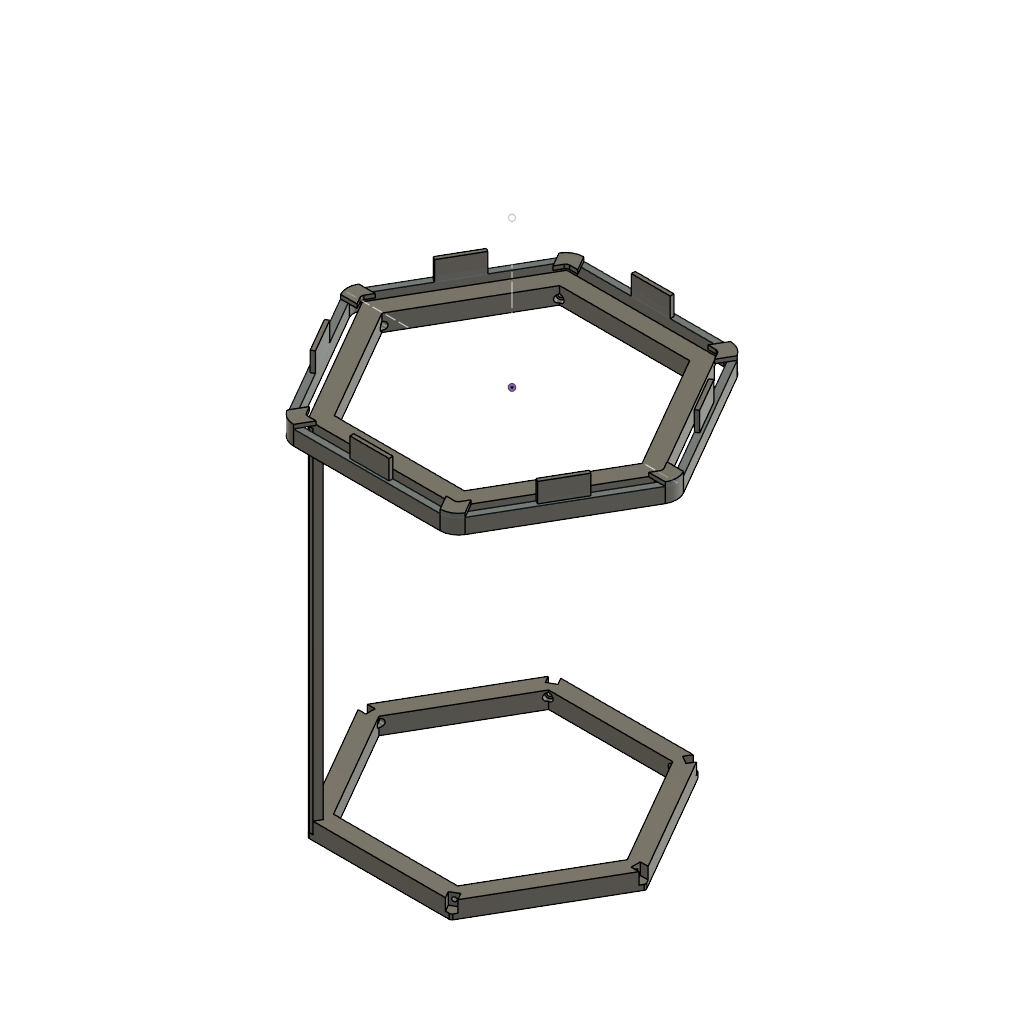
Transparent_PCB_Support (Autodesk Fusion 360 design; units mm, degrees)
Autodesk Fusion 360 part; units mm, degrees
sketch "Sketch1" plane through (0, 0, 0) normal (0, 1, 0) x (1, 0, 0) in component "TopHex"
  line L0 (0, 0) -> (114.9, 0)
  line L1 (114.9, 0) -> (172.35, 99.5063)
  line L2 (172.35, 99.5063) -> (114.9, 199.0126)
  line L3 (114.9, 199.0126) -> (0, 199.0126)
  line L4 (0, 199.0126) -> (-57.45, 99.5063)
  line L5 (-57.45, 99.5063) -> (0, 0)
  line L6 (-42.4389, 99.5063) -> (7.5056, 13)
  line L7 (7.5056, 13) -> (107.3944, 13)
  line L8 (107.3944, 13) -> (157.3389, 99.5063)
  line L9 (157.3389, 99.5063) -> (107.3944, 186.0126)
  line L10 (107.3944, 186.0126) -> (7.5056, 186.0126)
  line L11 (7.5056, 186.0126) -> (-42.4389, 99.5063)
  point P0 (57.45, 99.5063)
  dimension "d1" = 114.9
  dimension "d2" = -13
  constraint coincident L0.start L5.end
  measures "d1" distance of L0.start L0.end
extrude "Extrude1" add sketch "Sketch1" along normal blind 13 makes body 1 in component "TopHex"
ref_plane "WorkPlane1" through (114.9, 6.5, 0) normal (0.5, 0, 0.866025) x (0, 1, 0) in component "TopHex"
sketch "Sketch2" plane through (28.725, 0, 49.7532) normal (0.5, 0, 0.866025) x (0, 1, 0) in component "TopHex"
  line L0 (0, 0) -> (0, -99.5063) construction
  line L1 (0, -99.5063) -> (13, -99.5063) construction
  line L2 (13, -99.5063) -> (13, 0) construction
  line L3 (13, 0) -> (0, 0) construction
  line L4 (0, -99.5063) -> (0, -199.0126) construction
  line L5 (0, -199.0126) -> (13, -199.0126) construction
  line L6 (13, -199.0126) -> (13, -99.5063) construction
  line L7 (13, -99.5063) -> (0, -99.5063) construction
  line L8 (0, -99.5063) -> (9, -99.5063) construction
  line L9 (9, -103.0063) -> (0, -103.0063)
  line L10 (0, -103.0063) -> (0, -96.0063)
  line L11 (0, -96.0063) -> (9, -96.0063)
  line L12 (9, -96.0063) -> (9, -103.0063)
  line L13 (9, -103.0063) -> (0, -96.0063) construction
  line L14 (0, -103.0063) -> (9, -96.0063) construction
  point P0 (4.5, -99.5063)
  dimension "d6" = 9
  dimension "d7" = 7
  constraint coincident L0.end L1.start
  constraint perpendicular L4 L8
  constraint horizontal L9
  constraint perpendicular L9 L10
  constraint parallel L9 L11
  constraint parallel L10 L12
  constraint coincident L13 P0
  constraint coincident L14 P0
  constraint midpoint L8 P0
  constraint collinear L0 L10
  measures "d6" distance of L0.end L8.end
  measures "d7" distance of L9.end L10.end
extrude "Extrude2" cut sketch "Sketch2" against normal blind 8 bodies 1 in component "TopHex"
fillet "Fillet1" radius 2 1 edges at (114.9, 11, 0) on bodies 1 in component "TopHex"
sketch "Sketch3" plane through (24.725, 0, 42.825) normal (0.5, 0, 0.866025) x (0.866025, 0, -0.5) in component "TopHex"
  line L0 (96.0063, 9) -> (96.0063, 0)
  line L1 (96.0063, 0) -> (103.0063, 0)
  line L2 (103.0063, 0) -> (103.0063, 9)
  line L3 (103.0063, 9) -> (96.0063, 9)
  line L4 (96.0063, 9) -> (103.0063, 0) construction
  line L5 (96.0063, 0) -> (103.0063, 9) construction
  circle A0 centre (99.5063, 4.5) radius 1.6
  dimension "d12" = 3.2
  constraint coincident L0.start L3.end
  constraint coincident L1.end L2.start
  constraint coincident L0.end L1.start
  constraint coincident L2.end L3.start
  constraint midpoint L5 A0.centre
  measures "d12" diameter of A0
extrude "Extrude3" cut sketch "Sketch3" against normal blind 8.5 contours A0 bodies 1 in component "TopHex"
sketch "Sketch4" plane through (24.725, 0, 42.825) normal (0.5, 0, 0.866025) x (0.866025, 0, -0.5) in component "TopHex"
  circle A0 centre (99.5063, 4.5) radius 1.6
  line L0 (96.0063, 9) -> (96.0063, 0)
  line L1 (96.0063, 0) -> (103.0063, 0)
  line L2 (103.0063, 0) -> (103.0063, 9)
  line L3 (103.0063, 9) -> (96.0063, 9)
  circle A1 centre (99.5063, 4.5) radius 1.6 construction
  circle A2 centre (99.5063, 4.5) radius 3
  dimension "d15" = 6
  constraint concentric A1 A2
  measures "d15" diameter of A2
extrude "Extrude4" cut sketch "Sketch4" against normal blind 5 from surface at -4 contours A0 | A2 bodies 1 in component "TopHex"
sketch "Sketch5" plane through (0, 0, 0) normal (0, 1, 0) x (1, 0, 0) in component "TopHex"
  arc A0 (113.7453, 0) -> (115.4774, 1) centre (113.7453, 2) ccw construction
  line L0 (115.4774, 1) -> (172.35, 99.5063) construction
  line L1 (172.35, 99.5063) -> (114.9, 199.0126) construction
  line L2 (114.9, 199.0126) -> (0, 199.0126) construction
  line L3 (0, 199.0126) -> (-57.45, 99.5063) construction
  line L4 (-57.45, 99.5063) -> (0, 0) construction
  line L5 (0, 0) -> (113.7453, 0) construction
  line L6 (-42.4389, 99.5063) -> (7.5056, 186.0126) construction
  line L7 (7.5056, 186.0126) -> (107.3944, 186.0126) construction
  line L8 (107.3944, 186.0126) -> (157.3389, 99.5063) construction
  line L9 (157.3389, 99.5063) -> (107.3944, 13) construction
  line L10 (107.3944, 13) -> (7.5056, 13) construction
  line L11 (7.5056, 13) -> (-42.4389, 99.5063) construction
  line L12 (0, 0) -> (114.9, 199.0126) construction
  line L13 (0, 199.0126) -> (107.3944, 13) construction
  constraint coincident L4.end L5.start
  constraint coincident L1.end L2.start
  constraint coincident L2.end L3.start
  constraint coincident L9.end L10.start
ref_plane "WorkPlane2" through (57.45, 0, -99.5063) normal (0.5, 0, -0.866025) x (0, 1, 0) in component "TopHex"
sketch "Sketch6" plane through (57.45, 0, -99.5063) normal (0.5, 0, -0.866025) x (0, 1, 0) in component "TopHex"
  line L0 (0, 0) -> (113, 0)
  constraint coincident L0.start origin
  constraint horizontal L0
pattern_circular "C-Pattern1" count 6 over 360 about axis through (57.45, 0, -99.5063) along (0, 1, 0) of "Extrude2", "Extrude3", "Extrude4" in component "TopHex"
fillet "Fillet2" radius 2 5 edges at (172.35, 11, -99.5063) (114.9, 11, -199.0126) (0, 11, -199.0126) (-57.45, 11, -99.5063) (0, 11, 0) on bodies 1 in component "TopHex"
ref_plane "WorkPlane1" through (57.45, -265, -99.5063) normal (0, 1, 0) x (0, 0, 1) in component "BottomHex"
sketch "Sketch1 (2)" plane through (0, -265, 0) normal (0, 1, 0) x (1, 0, 0) in component "BottomHex"
  line L0 (0, 0) -> (109.9, 0)
  line L1 (109.9, 0) -> (164.85, 95.1762)
  line L2 (164.85, 95.1762) -> (109.9, 190.3524)
  line L3 (109.9, 190.3524) -> (0, 190.3524)
  line L4 (0, 190.3524) -> (-54.95, 95.1762)
  line L5 (-54.95, 95.1762) -> (0, 0)
  line L6 (7.2746, 12.6) -> (102.6254, 12.6)
  line L7 (102.6254, 12.6) -> (150.3008, 95.1762)
  line L8 (150.3008, 95.1762) -> (102.6254, 177.7524)
  line L9 (102.6254, 177.7524) -> (7.2746, 177.7524)
  line L10 (7.2746, 177.7524) -> (-40.4008, 95.1762)
  line L11 (-40.4008, 95.1762) -> (7.2746, 12.6)
  point P0 (54.95, 95.1762)
  dimension "d26" = 109.9
  dimension "d27" = -12.6
  constraint coincident L0.start L5.end
  measures "d26" distance of L0.start L0.end
extrude "Extrude1'" add sketch "Sketch1 (2)" along normal blind 13 separate body makes body 2 in component "BottomHex"
ref_plane "WorkPlane2" through (0, -258.5, 0) normal (-0.5, 0, 0.866025) x (0, 1, 0) in component "BottomHex"
sketch "Sketch2 (2)" plane through (0, 0, 0) normal (-0.5, 0, 0.866025) x (0, 1, 0) in component "BottomHex"
  line L0 (-265, 0) -> (-252, 0) construction
  line L1 (-265, 95.1762) -> (-265, 0) construction
  line L2 (-265, 0) -> (-252, 0) construction
  line L3 (-252, 0) -> (-252, 95.1762) construction
  line L4 (-252, 95.1762) -> (-265, 95.1762) construction
  line L5 (-265, 0) -> (-265, -95.1762) construction
  line L6 (-265, -95.1762) -> (-252, -95.1762) construction
  line L7 (-252, -95.1762) -> (-252, 0) construction
  line L8 (-252, 0) -> (-265, 0) construction
  line L9 (-252, 0) -> (-261, 0) construction
  line L10 (-252, -3.5) -> (-261, -3.5)
  line L11 (-261, -3.5) -> (-261, 3.5)
  line L12 (-261, 3.5) -> (-252, 3.5)
  line L13 (-252, 3.5) -> (-252, -3.5)
  line L14 (-252, -3.5) -> (-261, 3.5) construction
  line L15 (-261, -3.5) -> (-252, 3.5) construction
  point P0 (-256.5, 0)
  dimension "d31" = 9
  dimension "d32" = 9
  dimension "d33" = 7
  constraint coincident L0.end L2.end
  constraint perpendicular L3 L9
  constraint horizontal L10
  constraint perpendicular L10 L11
  constraint parallel L10 L12
  constraint parallel L11 L13
  constraint coincident L14 P0
  constraint coincident L15 P0
  constraint midpoint L9 P0
  measures "d31" distance of L0.end L9.end
  measures "d32" distance of L11.end L12.end
  measures "d33" distance of L10.end L11.end
extrude "Extrude2'" cut sketch "Sketch2 (2)" against normal blind 8 bodies 2 in component "BottomHex"
sketch "Sketch3 (2)" plane through (4, 0, -6.9282) normal (-0.5, 0, 0.866025) x (0.866025, 0, 0.5) in component "BottomHex"
  line L0 (-3.5, -252) -> (-3.5, -261)
  line L1 (-3.5, -261) -> (3.5, -261)
  line L2 (3.5, -261) -> (3.5, -252)
  line L3 (3.5, -252) -> (-3.5, -252)
  line L4 (-3.5, -261) -> (3.5, -252) construction
  line L5 (-3.5, -252) -> (3.5, -261) construction
  circle A0 centre (0, -256.5) radius 1.6
  dimension "d36" = 3.2
  constraint coincident L0.end L1.start
  constraint coincident L2.end L3.start
  constraint coincident L0.start L3.end
  constraint coincident L1.end L2.start
  constraint midpoint L4 A0.centre
  measures "d36" diameter of A0
extrude "Extrude3'" cut sketch "Sketch3 (2)" against normal blind 10 contours A0 bodies 2 in component "BottomHex"
sketch "Sketch4 (2)" plane through (4, 0, -6.9282) normal (-0.5, 0, 0.866025) x (0.866025, 0, 0.5) in component "BottomHex"
  circle A0 centre (0, -256.5) radius 1.6
  line L0 (-3.5, -252) -> (-3.5, -261)
  line L1 (-3.5, -261) -> (3.5, -261)
  line L2 (3.5, -261) -> (3.5, -252)
  line L3 (3.5, -252) -> (-3.5, -252)
  circle A1 centre (0, -256.5) radius 1.6 construction
  circle A2 centre (0, -256.5) radius 3
  dimension "d39" = 6
  constraint concentric A1 A2
  measures "d39" diameter of A2
extrude "Extrude4'" cut sketch "Sketch4 (2)" against normal blind 5 from surface at -4 contours A2 bodies 2 in component "BottomHex"
sketch "Sketch5 (2)" plane through (0, -252, 0) normal (0, 1, 0) x (-1, 0, 0) in component "BottomHex"
  line L0 (2.0207, -3.5) -> (-0.9689, -8.6782)
  line L1 (-0.9689, -8.6782) -> (-7.0311, -5.1782)
  line L2 (-7.0311, -5.1782) -> (-4.0415, 0)
  line L3 (-4.0415, 0) -> (-109.9, 0)
  line L4 (-109.9, 0) -> (-164.85, -95.1762)
  line L5 (-164.85, -95.1762) -> (-109.9, -190.3524)
  line L6 (-109.9, -190.3524) -> (0, -190.3524)
  line L7 (0, -190.3524) -> (54.95, -95.1762)
  line L8 (54.95, -95.1762) -> (2.0207, -3.5)
  line L9 (-7.2746, -12.6) -> (40.4008, -95.1762)
  line L10 (40.4008, -95.1762) -> (-7.2746, -177.7524)
  line L11 (-7.2746, -177.7524) -> (-102.6254, -177.7524)
  line L12 (-102.6254, -177.7524) -> (-150.3008, -95.1762)
  line L13 (-150.3008, -95.1762) -> (-102.6254, -12.6)
  line L14 (-102.6254, -12.6) -> (-7.2746, -12.6)
  line L15 (-7.2746, -12.6) -> (-102.6254, -177.7524) construction
  constraint coincident L9.start L14.end
  constraint coincident L11.end L12.start
ref_plane "WorkPlane3" through (54.95, -252, -95.1762) normal (0.5, 0, -0.866025) x (0, 1, 0) in component "BottomHex"
sketch "Sketch6 (2)" plane through (54.95, -252, -95.1762) normal (0.5, 0, -0.866025) x (0, 1, 0) in component "BottomHex"
  line L0 (0, 0) -> (115, 0)
  constraint coincident L0.start origin
  constraint horizontal L0
pattern_circular "C-Pattern1'" count 6 over 360 about axis through (54.95, -252, -95.1762) along (0, 1, 0) of "Extrude2'", "Extrude3'", "Extrude4'" in component "BottomHex"
fillet "Fillet1'" radius 2 6 edges at (0, -263, 0) (109.9, -263, 0) (164.85, -263, -95.1762) (109.9, -263, -190.3524) (0, -263, -190.3524) (-54.95, -263, -95.1762) on bodies 2 in component "BottomHex"
sketch "Sketch1 (3)" plane through (0, 9, 0) normal (0, -1, 0) x (1, 0, 0) in component "Connection"
  line L0 (-2.0207, -3.5) -> (0.9689, -8.6782)
  line L1 (0.9689, -8.6782) -> (7.0311, -5.1782)
  line L2 (7.0311, -5.1782) -> (4.0415, 0)
  line L3 (-2.0207, -3.5) -> (0.9689, -8.6782) construction
  line L4 (7.0311, -5.1782) -> (4.0415, 0) construction
  line L5 (0.9689, -8.6782) -> (7.0311, -5.1782) construction
  arc A0 (1.1547, 0) -> (-0.5774, -1) centre (1.1547, -2) ccw construction
  line L6 (1.1547, 0) -> (108.7453, 0) construction
  line L7 (-1.8764, -3.45) -> (1.0238, -8.4733)
  line L8 (1.0238, -8.4733) -> (6.8262, -5.1233)
  line L9 (6.8262, -5.1233) -> (3.926, -0.1)
  line L10 (-54.3726, -94.1762) -> (-0.5774, -1) construction
  arc A1 (1.1547, -0.1) -> (-0.4907, -1.05) centre (1.1547, -2) ccw
  line L11 (1.1547, -0.1) -> (3.926, -0.1)
  line L12 (-1.8764, -3.45) -> (-0.4907, -1.05)
  constraint coincident L0.start L3.start
  constraint coincident L0.end L1.start
  constraint coincident L1.end L2.start
  constraint coincident L2.end L4.end
  constraint concentric A0 A1
  constraint tangent A1 L11
extrude "Extrude1''" add sketch "Sketch1 (3)" along normal blind 270 separate body makes body 3 in component "Connection"
sketch "Sketch2 (3)" plane through (3.925, 0, -6.7983) normal (0.5, 0, -0.866025) x (-0.866025, 0, -0.5) in component "Connection"
  line L0 (3.35, 9) -> (-3.35, 9)
  line L1 (-3.35, 9) -> (-3.35, -261)
  line L2 (-3.35, -261) -> (3.35, -261)
  line L3 (3.35, -261) -> (3.35, 9)
  circle A0 centre (0, 4.5) radius 1.6 construction
  circle A1 centre (0, -256.5) radius 1.6 construction
  circle A2 centre (0, -256.5) radius 1.475
  circle A3 centre (0, 4.5) radius 1.475
  dimension "d52" = 2.95
  dimension "d53" = 2.95
  constraint concentric A1 A2
  constraint concentric A0 A3
  measures "d52" diameter of A2
  measures "d53" diameter of A3
extrude "Extrude2''" cut sketch "Sketch2 (3)" against normal blind 6 contours A2 | A3 bodies 3 in component "Connection"
ref_plane "WorkPlane1" through (57.45, 10, -99.5063) normal (0, 1, 0) x (0, 0, 1) in component "OutsideSupport"
sketch "Sketch1 (4)" plane through (0, 10, 0) normal (0, 1, 0) x (1, 0, 0) in component "OutsideSupport"
  arc A0 (-0.5774, 1) -> (1.1547, 0) centre (1.1547, 2) ccw construction
  line L0 (1.1547, 0) -> (113.7453, 0) construction
  arc A1 (113.7453, 0) -> (115.4774, 1) centre (113.7453, 2) ccw construction
  line L1 (115.4774, 1) -> (171.7726, 98.5063) construction
  arc A2 (171.7726, 98.5063) -> (171.7726, 100.5063) centre (170.0406, 99.5063) ccw construction
  line L2 (171.7726, 100.5063) -> (115.4774, 198.0126) construction
  arc A3 (115.4774, 198.0126) -> (113.7453, 199.0126) centre (113.7453, 197.0126) ccw construction
  line L3 (113.7453, 199.0126) -> (1.1547, 199.0126) construction
  arc A4 (1.1547, 199.0126) -> (-0.5774, 198.0126) centre (1.1547, 197.0126) ccw construction
  line L4 (-0.5774, 198.0126) -> (-56.8726, 100.5063) construction
  arc A5 (-56.8726, 100.5063) -> (-56.8726, 98.5063) centre (-55.1406, 99.5063) ccw construction
  line L5 (-56.8726, 98.5063) -> (-0.5774, 1) construction
  line L6 (-42.4389, 99.5063) -> (7.5056, 186.0126) construction
  line L7 (7.5056, 186.0126) -> (107.3944, 186.0126) construction
  line L8 (107.3944, 186.0126) -> (157.3389, 99.5063) construction
  line L9 (157.3389, 99.5063) -> (107.3944, 13) construction
  line L10 (107.3944, 13) -> (7.5056, 13) construction
  line L11 (7.5056, 13) -> (-42.4389, 99.5063) construction
  line L12 (121.5395, -2.5) -> (177.8348, 95.0063)
  arc A6 (177.8348, 95.0063) -> (177.8348, 104.0063) centre (170.0406, 99.5063) ccw
  line L13 (177.8348, 104.0063) -> (121.5395, 201.5126)
  arc A7 (121.5395, 201.5126) -> (113.7453, 206.0126) centre (113.7453, 197.0126) ccw
  line L14 (113.7453, 206.0126) -> (1.1547, 206.0126)
  arc A8 (1.1547, 206.0126) -> (-6.6395, 201.5126) centre (1.1547, 197.0126) ccw
  line L15 (-6.6395, 201.5126) -> (-62.9348, 104.0063)
  arc A9 (-62.9348, 104.0063) -> (-62.9348, 95.0063) centre (-55.1406, 99.5063) ccw
  line L16 (-62.9348, 95.0063) -> (-6.6395, -2.5)
  arc A10 (-6.6395, -2.5) -> (1.1547, -7) centre (1.1547, 2) ccw
  line L17 (1.1547, -7) -> (113.7453, -7)
  arc A11 (113.7453, -7) -> (121.5395, -2.5) centre (113.7453, 2) ccw
  line L18 (125.8697, -5) -> (182.165, 92.5063)
  arc A12 (182.165, 92.5063) -> (182.165, 106.5063) centre (170.0406, 99.5063) ccw
  line L19 (182.165, 106.5063) -> (125.8697, 204.0126)
  arc A13 (125.8697, 204.0126) -> (113.7453, 211.0126) centre (113.7453, 197.0126) ccw
  line L20 (113.7453, 211.0126) -> (1.1547, 211.0126)
  arc A14 (1.1547, 211.0126) -> (-10.9697, 204.0126) centre (1.1547, 197.0126) ccw
  line L21 (-10.9697, 204.0126) -> (-67.265, 106.5063)
  arc A15 (-67.265, 106.5063) -> (-67.265, 92.5063) centre (-55.1406, 99.5063) ccw
  line L22 (-67.265, 92.5063) -> (-10.9697, -5)
  arc A16 (-10.9697, -5) -> (1.1547, -12) centre (1.1547, 2) ccw
  line L23 (1.1547, -12) -> (113.7453, -12)
  arc A17 (113.7453, -12) -> (125.8697, -5) centre (113.7453, 2) ccw
  dimension "d57" = 7
  dimension "d58" = 12
extrude "Extrude1'''" add sketch "Sketch1 (4)" against normal blind 8 separate body makes body 4 in component "OutsideSupport"
sketch "Sketch2 (4)" plane through (0, 10, 0) normal (0, 1, 0) x (-1, 0, 0) in component "OutsideSupport"
  arc A0 (-113.7453, 7) -> (-121.5395, 2.5) centre (-113.7453, -2) ccw
  line L0 (-113.7453, 7) -> (-1.1547, 7)
  arc A1 (6.6395, 2.5) -> (-1.1547, 7) centre (-1.1547, -2) ccw
  line L1 (6.6395, 2.5) -> (62.9348, -95.0063)
  arc A2 (62.9348, -104.0063) -> (62.9348, -95.0063) centre (55.1406, -99.5063) ccw
  line L2 (62.9348, -104.0063) -> (6.6395, -201.5126)
  arc A3 (-1.1547, -206.0126) -> (6.6395, -201.5126) centre (-1.1547, -197.0126) ccw
  line L3 (-1.1547, -206.0126) -> (-113.7453, -206.0126)
  arc A4 (-121.5395, -201.5126) -> (-113.7453, -206.0126) centre (-113.7453, -197.0126) ccw
  line L4 (-121.5395, -201.5126) -> (-177.8348, -104.0063)
  arc A5 (-177.8348, -95.0063) -> (-177.8348, -104.0063) centre (-170.0406, -99.5063) ccw
  line L5 (-177.8348, -95.0063) -> (-121.5395, 2.5)
  arc A6 (-113.7453, 12) -> (-125.8697, 5) centre (-113.7453, -2) ccw
  line L6 (-125.8697, 5) -> (-182.165, -92.5063)
  arc A7 (-182.165, -92.5063) -> (-182.165, -106.5063) centre (-170.0406, -99.5063) ccw
  line L7 (-182.165, -106.5063) -> (-125.8697, -204.0126)
  arc A8 (-125.8697, -204.0126) -> (-113.7453, -211.0126) centre (-113.7453, -197.0126) ccw
  line L8 (-113.7453, -211.0126) -> (-1.1547, -211.0126)
  arc A9 (-1.1547, -211.0126) -> (10.9697, -204.0126) centre (-1.1547, -197.0126) ccw
  line L9 (10.9697, -204.0126) -> (67.265, -106.5063)
  arc A10 (67.265, -106.5063) -> (67.265, -92.5063) centre (55.1406, -99.5063) ccw
  line L10 (67.265, -92.5063) -> (10.9697, 5)
  arc A11 (10.9697, 5) -> (-1.1547, 12) centre (-1.1547, -2) ccw
  line L11 (-1.1547, 12) -> (-113.7453, 12)
  line L12 (6.6395, 2.5) -> (62.9348, -95.0063) construction
  arc A12 (64.6669, -105.0063) -> (64.6669, -94.0063) centre (55.1406, -99.5063) ccw
  line L13 (8.3716, 3.5) -> (64.6669, -94.0063)
  arc A13 (8.3716, 3.5) -> (-1.1547, 9) centre (-1.1547, -2) ccw
  line L14 (-113.7453, 9) -> (-1.1547, 9)
  arc A14 (-113.7453, 9) -> (-123.2716, 3.5) centre (-113.7453, -2) ccw
  line L15 (-179.5669, -94.0063) -> (-123.2716, 3.5)
  arc A15 (-179.5669, -94.0063) -> (-179.5669, -105.0063) centre (-170.0406, -99.5063) ccw
  line L16 (-123.2716, -202.5126) -> (-179.5669, -105.0063)
  arc A16 (-123.2716, -202.5126) -> (-113.7453, -208.0126) centre (-113.7453, -197.0126) ccw
  line L17 (-1.1547, -208.0126) -> (-113.7453, -208.0126)
  arc A17 (-1.1547, -208.0126) -> (8.3716, -202.5126) centre (-1.1547, -197.0126) ccw
  line L18 (64.6669, -105.0063) -> (8.3716, -202.5126)
  dimension "d61" = -2
extrude "Extrude2'''" add sketch "Sketch2 (4)" along normal blind 3.5 contours A6 L6 A7 L7 A8 L8 A9 L9 A10 L10 A11 L11 | A12 L13 A13 L14 A14 L15 A15 L16 A16 L17 A17 L18 bodies 4 in component "OutsideSupport"
sketch "Sketch3 (3)" plane through (0, 13.5, 0) normal (0, 1, 0) x (-1, 0, 0) in component "OutsideSupport"
  line L0 (-1.1547, 12) -> (-113.7453, 12)
  arc A0 (-113.7453, 12) -> (-125.8697, 5) centre (-113.7453, -2) ccw
  line L1 (-125.8697, 5) -> (-182.165, -92.5063)
  arc A1 (-182.165, -92.5063) -> (-182.165, -106.5063) centre (-170.0406, -99.5063) ccw
  line L2 (-182.165, -106.5063) -> (-125.8697, -204.0126)
  arc A2 (-125.8697, -204.0126) -> (-113.7453, -211.0126) centre (-113.7453, -197.0126) ccw
  line L3 (-113.7453, -211.0126) -> (-1.1547, -211.0126)
  arc A3 (-1.1547, -211.0126) -> (10.9697, -204.0126) centre (-1.1547, -197.0126) ccw
  line L4 (10.9697, -204.0126) -> (67.265, -106.5063)
  arc A4 (67.265, -106.5063) -> (67.265, -92.5063) centre (55.1406, -99.5063) ccw
  line L5 (67.265, -92.5063) -> (10.9697, 5)
  arc A5 (10.9697, 5) -> (-1.1547, 12) centre (-1.1547, -2) ccw
  arc A6 (0.5774, -1) -> (-1.1547, 0) centre (-1.1547, -2) ccw construction
  line L6 (-1.1547, 0) -> (-113.7453, 0) construction
  arc A7 (-113.7453, 0) -> (-115.4774, -1) centre (-113.7453, -2) ccw construction
  line L7 (-115.4774, -1) -> (-171.7726, -98.5063) construction
  arc A8 (-171.7726, -98.5063) -> (-171.7726, -100.5063) centre (-170.0406, -99.5063) ccw construction
  line L8 (-171.7726, -100.5063) -> (-115.4774, -198.0126) construction
  arc A9 (-115.4774, -198.0126) -> (-113.7453, -199.0126) centre (-113.7453, -197.0126) ccw construction
  line L9 (-113.7453, -199.0126) -> (-1.1547, -199.0126) construction
  arc A10 (-1.1547, -199.0126) -> (0.5774, -198.0126) centre (-1.1547, -197.0126) ccw construction
  line L10 (0.5774, -198.0126) -> (56.8726, -100.5063) construction
  arc A11 (56.8726, -100.5063) -> (56.8726, -98.5063) centre (55.1406, -99.5063) ccw construction
  line L11 (56.8726, -98.5063) -> (0.5774, -1) construction
  line L12 (42.4389, -99.5063) -> (-7.5056, -186.0126) construction
  line L13 (-7.5056, -186.0126) -> (-107.3944, -186.0126) construction
  line L14 (-107.3944, -186.0126) -> (-157.3389, -99.5063) construction
  line L15 (-157.3389, -99.5063) -> (-107.3944, -13) construction
  line L16 (-107.3944, -13) -> (-7.5056, -13) construction
  line L17 (-7.5056, -13) -> (42.4389, -99.5063) construction
  line L18 (41.2842, -99.5063) -> (-8.0829, -185.0126)
  line L19 (-8.0829, -185.0126) -> (-106.8171, -185.0126)
  line L20 (-106.8171, -185.0126) -> (-156.1842, -99.5063)
  line L21 (-156.1842, -99.5063) -> (-106.8171, -14)
  line L22 (-106.8171, -14) -> (-8.0829, -14)
  line L23 (-8.0829, -14) -> (41.2842, -99.5063)
  arc A12 (-113.7453, 7) -> (-121.5395, 2.5) centre (-113.7453, -2) ccw
  line L24 (-121.5395, 2.5) -> (-177.8348, -95.0063)
  arc A13 (-177.8348, -95.0063) -> (-177.8348, -104.0063) centre (-170.0406, -99.5063) ccw
  line L25 (-177.8348, -104.0063) -> (-121.5395, -201.5126)
  arc A14 (-121.5395, -201.5126) -> (-113.7453, -206.0126) centre (-113.7453, -197.0126) ccw
  line L26 (-113.7453, -206.0126) -> (-1.1547, -206.0126)
  arc A15 (-1.1547, -206.0126) -> (6.6395, -201.5126) centre (-1.1547, -197.0126) ccw
  line L27 (6.6395, -201.5126) -> (62.9348, -104.0063)
  arc A16 (62.9348, -104.0063) -> (62.9348, -95.0063) centre (55.1406, -99.5063) ccw
  line L28 (62.9348, -95.0063) -> (6.6395, 2.5)
  arc A17 (6.6395, 2.5) -> (-1.1547, 7) centre (-1.1547, -2) ccw
  line L29 (-1.1547, 7) -> (-113.7453, 7)
  arc A18 (-113.7453, 12) -> (-125.8697, 5) centre (-113.7453, -2) ccw
  line L30 (-113.7453, 12) -> (-1.1547, 12)
  arc A19 (10.9697, 5) -> (-1.1547, 12) centre (-1.1547, -2) ccw
  line L31 (10.9697, 5) -> (67.265, -92.5063)
  arc A20 (67.265, -106.5063) -> (67.265, -92.5063) centre (55.1406, -99.5063) ccw
  line L32 (67.265, -106.5063) -> (10.9697, -204.0126)
  arc A21 (-1.1547, -211.0126) -> (10.9697, -204.0126) centre (-1.1547, -197.0126) ccw
  line L33 (-1.1547, -211.0126) -> (-113.7453, -211.0126)
  arc A22 (-125.8697, -204.0126) -> (-113.7453, -211.0126) centre (-113.7453, -197.0126) ccw
  line L34 (-125.8697, -204.0126) -> (-182.165, -106.5063)
  arc A23 (-182.165, -92.5063) -> (-182.165, -106.5063) centre (-170.0406, -99.5063) ccw
  line L35 (-182.165, -92.5063) -> (-125.8697, 5)
  arc A24 (-121.5395, -201.5126) -> (-113.7453, -206.0126) centre (-113.7453, -197.0126) ccw
  line L36 (-121.5395, -201.5126) -> (-177.8348, -104.0063)
  arc A25 (-177.8348, -95.0063) -> (-177.8348, -104.0063) centre (-170.0406, -99.5063) ccw
  line L37 (-177.8348, -95.0063) -> (-121.5395, 2.5)
  arc A26 (-113.7453, 7) -> (-121.5395, 2.5) centre (-113.7453, -2) ccw
  line L38 (-113.7453, 7) -> (-1.1547, 7)
  arc A27 (6.6395, 2.5) -> (-1.1547, 7) centre (-1.1547, -2) ccw
  line L39 (6.6395, 2.5) -> (62.9348, -95.0063)
  arc A28 (62.9348, -104.0063) -> (62.9348, -95.0063) centre (55.1406, -99.5063) ccw
  line L40 (62.9348, -104.0063) -> (6.6395, -201.5126)
  arc A29 (-1.1547, -206.0126) -> (6.6395, -201.5126) centre (-1.1547, -197.0126) ccw
  line L41 (-1.1547, -206.0126) -> (-113.7453, -206.0126)
  line L42 (-0.1547, -0.2679) -> (5.8453, 10.1244)
  line L43 (-1.1547, 12) -> (-8.0829, 0)
  line L44 (-116.3434, -0.5) -> (-172.6387, -98.0063)
  arc A30 (-172.6387, -98.0063) -> (-172.6387, -101.0063) centre (-170.0406, -99.5063) ccw
  line L45 (-172.6387, -101.0063) -> (-116.3434, -198.5126)
  arc A31 (-116.3434, -198.5126) -> (-113.7453, -200.0126) centre (-113.7453, -197.0126) ccw
  line L46 (-113.7453, -200.0126) -> (-1.1547, -200.0126)
  arc A32 (-1.1547, -200.0126) -> (1.4434, -198.5126) centre (-1.1547, -197.0126) ccw
  line L47 (1.4434, -198.5126) -> (57.7387, -101.0063)
  arc A33 (57.7387, -101.0063) -> (57.7387, -98.0063) centre (55.1406, -99.5063) ccw
  line L48 (57.7387, -98.0063) -> (1.4434, -0.5)
  arc A34 (1.4434, -0.5) -> (-1.1547, 1) centre (-1.1547, -2) ccw
  line L49 (-1.1547, 1) -> (-113.7453, 1)
  arc A35 (-113.7453, 1) -> (-116.3434, -0.5) centre (-113.7453, -2) ccw
  line L50 (10.9697, 5) -> (4.0415, -7)
  dimension "d64" = 1
  dimension "d74" = 1
  constraint midpoint A6 L42.start
  constraint midpoint A19 L42.end
  constraint coincident L0.start A5.end
  constraint coincident L6 L43.end
  constraint parallel L42 L43
  constraint symmetric L42 L0.start L5.end
  constraint symmetric L42 L43.end L50.end
extrude "Extrude3''" add sketch "Sketch3 (3)" along normal blind 3 contours A5 A17 L29 A19 L38 A27 L42 L43 | A5 L28 A17 A19 A27 L39 L42 L50 | A17 L29 L38 A27 L42 L43 A34 L49 | L28 A17 A27 L39 L42 L48 A34 L50 bodies 4 in component "OutsideSupport"
sketch "Sketch4 (3)" plane through (0, 13.5, 0) normal (0, 1, 0) x (-1, 0, 0) in component "OutsideSupport"
  arc A0 (0.5774, -1) -> (-1.1547, 0) centre (-1.1547, -2) ccw construction
  line L0 (-1.1547, 0) -> (-113.7453, 0) construction
  arc A1 (-113.7453, 0) -> (-115.4774, -1) centre (-113.7453, -2) ccw construction
  line L1 (-115.4774, -1) -> (-171.7726, -98.5063) construction
  arc A2 (-171.7726, -98.5063) -> (-171.7726, -100.5063) centre (-170.0406, -99.5063) ccw construction
  line L2 (-171.7726, -100.5063) -> (-115.4774, -198.0126) construction
  arc A3 (-115.4774, -198.0126) -> (-113.7453, -199.0126) centre (-113.7453, -197.0126) ccw construction
  line L3 (-113.7453, -199.0126) -> (-1.1547, -199.0126) construction
  arc A4 (-1.1547, -199.0126) -> (0.5774, -198.0126) centre (-1.1547, -197.0126) ccw construction
  line L4 (0.5774, -198.0126) -> (56.8726, -100.5063) construction
  arc A5 (56.8726, -100.5063) -> (56.8726, -98.5063) centre (55.1406, -99.5063) ccw construction
  line L5 (56.8726, -98.5063) -> (0.5774, -1) construction
  line L6 (42.4389, -99.5063) -> (-7.5056, -186.0126) construction
  line L7 (-7.5056, -186.0126) -> (-107.3944, -186.0126) construction
  line L8 (-107.3944, -186.0126) -> (-157.3389, -99.5063) construction
  line L9 (-157.3389, -99.5063) -> (-107.3944, -13) construction
  line L10 (-107.3944, -13) -> (-7.5056, -13) construction
  line L11 (-7.5056, -13) -> (42.4389, -99.5063) construction
  line L12 (-57.45, -13) -> (-57.45, 10) construction
  line L13 (-42.45, 7) -> (-57.45, 7)
  line L14 (-57.45, 7) -> (-57.45, 10)
  line L15 (-57.45, 10) -> (-42.45, 10)
  line L16 (-42.45, 10) -> (-42.45, 7)
  line L17 (-72.45, 7) -> (-57.45, 7)
  line L18 (-72.45, 10) -> (-72.45, 7)
  line L19 (-57.45, 10) -> (-72.45, 10)
  line L20 (8.0829, 0) -> (62.9348, -95.0063)
  line L21 (-113.7453, 7) -> (-4.0415, 7)
  line L22 (-4.0415, 7) -> (-1.1547, 12)
  line L23 (10.9697, 5) -> (8.0829, 0)
  arc A6 (62.9348, -104.0063) -> (62.9348, -95.0063) centre (55.1406, -99.5063) ccw
  line L24 (62.9348, -104.0063) -> (6.6395, -201.5126)
  arc A7 (-1.1547, -206.0126) -> (6.6395, -201.5126) centre (-1.1547, -197.0126) ccw
  line L25 (-1.1547, -206.0126) -> (-113.7453, -206.0126)
  arc A8 (-121.5395, -201.5126) -> (-113.7453, -206.0126) centre (-113.7453, -197.0126) ccw
  line L26 (-121.5395, -201.5126) -> (-177.8348, -104.0063)
  arc A9 (-177.8348, -95.0063) -> (-177.8348, -104.0063) centre (-170.0406, -99.5063) ccw
  line L27 (-177.8348, -95.0063) -> (-121.5395, 2.5)
  arc A10 (-113.7453, 7) -> (-121.5395, 2.5) centre (-113.7453, -2) ccw
  line L28 (-1.1547, 12) -> (-113.7453, 12)
  arc A11 (-113.7453, 12) -> (-125.8697, 5) centre (-113.7453, -2) ccw
  line L29 (-125.8697, 5) -> (-182.165, -92.5063)
  arc A12 (-182.165, -92.5063) -> (-182.165, -106.5063) centre (-170.0406, -99.5063) ccw
  line L30 (-182.165, -106.5063) -> (-125.8697, -204.0126)
  arc A13 (-125.8697, -204.0126) -> (-113.7453, -211.0126) centre (-113.7453, -197.0126) ccw
  line L31 (-113.7453, -211.0126) -> (-1.1547, -211.0126)
  arc A14 (-1.1547, -211.0126) -> (10.9697, -204.0126) centre (-1.1547, -197.0126) ccw
  line L32 (10.9697, -204.0126) -> (67.265, -106.5063)
  arc A15 (67.265, -106.5063) -> (67.265, -92.5063) centre (55.1406, -99.5063) ccw
  line L33 (67.265, -92.5063) -> (10.9697, 5)
  dimension "d70" = 15
  dimension "d71" = 3
  constraint midpoint L10 L12.start
  constraint horizontal L13
  constraint vertical L14
  constraint horizontal L15
  constraint vertical L16
  constraint collinear L12 L14
  constraint symmetric L12 L13.start L17.start
  constraint symmetric L12 L13.end L14.start
  constraint symmetric L12 L14.end L15.start
  constraint symmetric L12 L15.end L18.start
  constraint collinear L17 L21
  measures "d70" distance of L13.start L13.end
  measures "d71" distance of L13 L15
extrude "Extrude5" add sketch "Sketch4 (3)" along normal blind 15 contours L13 L14 L15 L16 L21 | L14 L17 L18 L19 L21 bodies 4 in component "OutsideSupport"
sketch "Sketch5 (3)" plane through (0, 13.5, 0) normal (0, 1, 0) x (-1, 0, 0) in component "OutsideSupport"
  line L0 (-72.45, 7) -> (-72.45, 10)
  line L1 (-72.45, 10) -> (-42.45, 10)
  line L2 (-42.45, 10) -> (-42.45, 7)
  line L3 (-42.45, 7) -> (-4.0415, 7)
  line L4 (-4.0415, 7) -> (-1.1547, 12)
  line L5 (-1.1547, 12) -> (-113.7453, 12)
  arc A0 (-113.7453, 12) -> (-125.8697, 5) centre (-113.7453, -2) ccw
  line L6 (-125.8697, 5) -> (-182.165, -92.5063)
  arc A1 (-182.165, -92.5063) -> (-182.165, -106.5063) centre (-170.0406, -99.5063) ccw
  line L7 (-182.165, -106.5063) -> (-125.8697, -204.0126)
  arc A2 (-125.8697, -204.0126) -> (-113.7453, -211.0126) centre (-113.7453, -197.0126) ccw
  line L8 (-113.7453, -211.0126) -> (-1.1547, -211.0126)
  arc A3 (-1.1547, -211.0126) -> (10.9697, -204.0126) centre (-1.1547, -197.0126) ccw
  line L9 (10.9697, -204.0126) -> (67.265, -106.5063)
  arc A4 (67.265, -106.5063) -> (67.265, -92.5063) centre (55.1406, -99.5063) ccw
  line L10 (67.265, -92.5063) -> (10.9697, 5)
  line L11 (10.9697, 5) -> (8.0829, 0)
  line L12 (8.0829, 0) -> (62.9348, -95.0063)
  arc A5 (62.9348, -104.0063) -> (62.9348, -95.0063) centre (55.1406, -99.5063) ccw
  line L13 (62.9348, -104.0063) -> (6.6395, -201.5126)
  arc A6 (-1.1547, -206.0126) -> (6.6395, -201.5126) centre (-1.1547, -197.0126) ccw
  line L14 (-1.1547, -206.0126) -> (-113.7453, -206.0126)
  arc A7 (-121.5395, -201.5126) -> (-113.7453, -206.0126) centre (-113.7453, -197.0126) ccw
  line L15 (-121.5395, -201.5126) -> (-177.8348, -104.0063)
  arc A8 (-177.8348, -95.0063) -> (-177.8348, -104.0063) centre (-170.0406, -99.5063) ccw
  line L16 (-177.8348, -95.0063) -> (-121.5395, 2.5)
  arc A9 (-113.7453, 7) -> (-121.5395, 2.5) centre (-113.7453, -2) ccw
  line L17 (-113.7453, 7) -> (-72.45, 7)
  line L18 (69.1406, -99.5063) -> (-184.0406, -99.5063) construction
  point P0 (-57.45, -99.5063)
  constraint midpoint A4 L18.start
  constraint midpoint A1 L18.end
  constraint midpoint L18 P0
ref_plane "WorkPlane2" through (57.45, 13.5, -99.5063) normal (1, 0, 0) x (0, 1, 0) in component "OutsideSupport"
sketch "Sketch6 (3)" plane through (57.45, 13.5, -99.5063) normal (1, 0, 0) x (0, 1, 0) in component "OutsideSupport"
  line L0 (0, 0) -> (112.7524, 0)
  constraint coincident L0.start origin
  constraint horizontal L0
pattern_circular "C-Pattern1''" count 6 over 360 about axis through (57.45, 13.5, -99.5063) along (0, 1, 0) of "Extrude3''", "Extrude5" in component "OutsideSupport"
component "TopHex" placed x (1, 0, 0) y (0, 1, 0) z (0, 0, 1) at (0, 0, 0)
component "BottomHex" placed x (1, 0, 0) y (0, 1, 0) z (0, 0, 1) at (0, 0, 0)
component "Connection" placed x (1, 0, 0) y (0, 1, 0) z (0, 0, 1) at (0, 0, 0)
component "OutsideSupport" placed x (1, 0, 0) y (0, 1, 0) z (0, 0, 1) at (0, 0, 0)
equation "d25 = -150 mm - 128 mm"
equation "d58 = 5 mm + d57"
